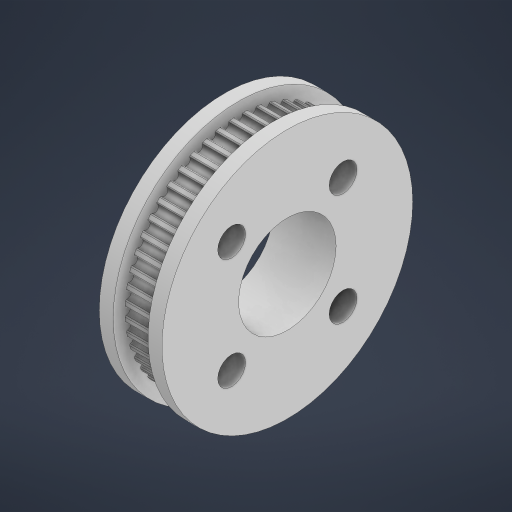
# Autodesk Inventor part: GT2 Pulley
Saved by Autodesk Inventor 2024 (Build 280153000, 153)
## iProperties
Created: 2023-10-25
Part Number: GT2 Pulley
Material: Generic
Document SubType Name: Modeling
Designer: avsar
Density: 1 g/cm^3
Appearance: Default
Author: avsar
Autodesk Inventor part; units mm, degrees
ref_plane "YZ Plane" through (0, 0, 0) normal (1, 0, 0) x (0, 1, 0)
ref_plane "XZ Plane" through (0, 0, 0) normal (0, 1, 0) x (-1, 0, 0)
ref_plane "XY Plane" through (0, 0, 0) normal (0, 0, 1) x (1, 0, 0)
sketch "Sketch1" plane through (0, 0, 0) normal (1, 0, 0) x (0, 1, 0)
  circle A0 centre (0, 0) radius 16.2981 construction
  circle A1 centre (0, 0) radius 15.5481 construction
  line L0 (0, 0) -> (16.2981, 0) construction
  line L1 (0, 0) -> (0, -16.2981) construction
  circle A2 centre (16.1031, 0) radius 0.555 construction
  line L2 (0, 0) -> (16.1793, -1.9645) construction
  circle A3 centre (15.9857, -1.941) radius 0.555 construction
  circle A4 centre (16.1327, -0.7044) radius 0.15 construction
  circle A5 centre (16.1, -1.2453) radius 0.15 construction
  arc A6 (15.5481, 0) -> (16.1264, -0.5545) centre (16.1031, 0) ccw
  arc A7 (16.2826, -0.7109) -> (16.1264, -0.5545) centre (16.1327, -0.7044) ccw
  arc A8 (16.2496, -1.2569) -> (16.2826, -0.7109) centre (0, 0) ccw
  arc A9 (16.0757, -1.3934) -> (16.2496, -1.2569) centre (16.1, -1.2453) ccw
  arc A10 (16.0757, -1.3934) -> (15.4348, -1.8741) centre (15.9857, -1.941) ccw
  arc A11 (15.4348, -1.8741) -> (15.5481, 0) centre (0, 0) ccw
  dimension "d0" = 32.5962
  dimension "d1" = -0.75
  dimension "d2" = 1.11
  dimension "d4" = 83.077
  dimension "d5" = 0.3
  constraints: 25 point on circle, 12 centre point, 8 equal radius, 8 tangent, 6 end point, 4 point on line, 1 coincident, 1 concentric, 1 horizontal, 1 perpendicular
  measures "d0" diameter of A0
  measures "d1" radial gap between concentric circles of A0 A1
  measures "d2" diameter of A2
  measures "d4" angle of L1 L2
  measures "d5" diameter of A4
extrude "Extrusion1" add sketch "Sketch1" along normal mid plane 5
pattern_circular "Circular Pattern1" count 52 over 360 about axis through (-10, 0, 0) along (1, 0, 0) of "Extrusion1"
sketch "Sketch2" plane through (0, 0, 0) normal (1, 0, 0) x (0, 1, 0)
  arc A0 (15.4348, 1.8741) -> (16.0757, 1.3934) centre (15.9857, 1.941) ccw projected
  circle A1 centre (0, 0) radius 15.5481
  constraints: 1 coincident, 3 other
extrude "Extrusion2" add sketch "Sketch2" along normal mid plane 5
sketch "Sketch5" plane through (2.5, 0, 0) normal (1, 0, 0) x (0, 0, -1)
  circle A0 centre (0, 0) radius 18
  dimension "d17" = 36
  constraints: 1 centre point, 1 coincident
  measures "d17" diameter of A0
extrude "Extrusion4" add sketch "Sketch5" along normal blind 2
sketch "Sketch10" plane through (-2.5, 0, 0) normal (-1, 0, 0) x (0, 0, 1)
  circle A0 centre (0, 0) radius 18 projected
extrude "Extrusion8" add sketch "Sketch10" along normal blind 2
sketch "Sketch11" plane through (-4.5, 0, 0) normal (-1, 0, 0) x (0, 0, 1)
  circle A0 centre (0, 0) radius 7
  circle A1 centre (-8, 8) radius 2
  circle A2 centre (-8, -8) radius 2
  circle A3 centre (8, -8) radius 2
  circle A4 centre (8, 8) radius 2
  dimension "d40" = 14
  dimension "d41" = 4
  dimension "d42" = 8
  dimension "d43" = 8
  dimension "d46" = 360
  constraints: 5 centre point, 1 coincident, 9 other
  measures "d40" diameter of A0
  measures "d41" diameter of A1
  measures "d42" horizontal distance of point (0, 0) A1.centre
  measures "d43" horizontal distance of point (0, 0) A1.centre
extrude "Extrusion9" cut sketch "Sketch11" against normal through all
equation "\"d0\" = OD_"
equation "\"d1\" = H_"
equation "\"d2\" = BTD_"
equation "\"d4\" = TH_"
equation "\"d5\" = PTR_"
equation "\"d6\" = EX_"
equation "\"d11\" = EX_"
equation "\"U_\" = 0.254"
equation "\"H_\" = -0.75"
equation "\"P_\" = 2"
equation "\"BTD_\" = 1.11"
equation "\"PTR_\" = 0.3"
equation "\"EX_\" = 5"
equation "\"OD_\" = PD_ - 2 * U_"
equation "\"TH_\" = 83.076923deg"
equation "\"PD_\" = 33.104228"
body "Solid1"
